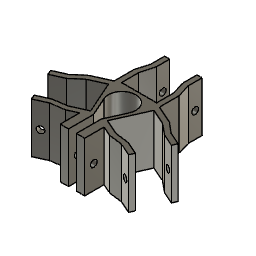
Battery Mount v1 (Autodesk Fusion 360 design; units mm, degrees)
Autodesk Fusion 360 part; units mm, degrees
note: some values were not read from the file. Set by a fixed rule: which sketch regions a step uses.
sketch "Sketch1" plane through (0, 0, 0) normal (0, 0, 1) x (1, 0, 0)
  line L0 (13.272, -15.3179) -> (7.3523, -12.6772)
  line L1 (22.727, -13.5264) -> (30.3778, -16.9328)
  line L2 (-18.8579, 11.9823) -> (-24.3388, 9.542)
  line L3 (-29.3341, 1.3169) -> (-26.7926, 3.4917)
  line L4 (10.5494, 15.7225) -> (10.5494, 25.9225)
  line L5 (-10.5507, 13.6692) -> (-12.6022, 13.6677)
  line L6 (-8.2853, 34.3148) -> (-10.558, 25.9259)
  line L7 (-22.9605, 6.8087) -> (-29.3341, 1.3169)
  line L8 (7.4982, 2.1403) -> (12.6022, 13.6692)
  line L9 (38.2942, 0.8476) -> (30.7617, 4.2012)
  line L10 (-18.8387, 11.9858) -> (-18.8579, 11.9823)
  line L11 (-13.6423, 10.9575) -> (-22.9605, 6.8087)
  line L12 (9.0778, 30.7724) -> (10.5494, 25.9225)
  line L13 (-13.6111, 26.0626) -> (-11.3383, 34.1084)
  line L14 (-36.985, -2.0895) -> (-29.3341, 1.3169)
  line L15 (37.0524, -1.9415) -> (29.7085, 1.3282)
  line L16 (30.7617, 4.2012) -> (24.3359, 9.5501)
  line L17 (-2.349, -24.3308) -> (-7.349, -24.3308)
  line L18 (13.607, 26.0699) -> (11.1789, 34.1274)
  line L19 (-24.3388, 9.542) -> (-30.7121, 4.0465)
  line L20 (-11.3383, 34.1084) -> (-13.6111, 26.0626)
  line L21 (-22.9605, 6.8087) -> (-13.6423, 10.9575)
  line L22 (30.3778, -16.9328) -> (29.1361, -19.7219)
  line L23 (-8.2853, 42.3537) -> (-11.3383, 42.3537)
  line L24 (37.0524, -1.9415) -> (38.2942, 0.8476)
  line L25 (2.3523, -24.3308) -> (7.3523, -24.3308)
  line L26 (-22.9665, -13.8111) -> (-14.3785, -12.4752)
  line L27 (-11.3383, 42.3537) -> (-8.2853, 42.3537)
  line L28 (-14.3785, -12.4752) -> (-22.9665, -13.8111)
  line L29 (-8.2853, 42.3537) -> (-8.2853, 34.3148)
  line L30 (7.3523, -12.6772) -> (7.3523, -24.3308)
  line L31 (8.1248, 33.9788) -> (9.0778, 30.7724)
  line L32 (11.1789, 34.1274) -> (13.607, 26.0699)
  line L33 (-2.349, -24.3308) -> (-2.349, -9.3308)
  line L34 (8.1248, 33.9788) -> (8.1248, 42.3537)
  line L35 (10.5494, 25.9225) -> (8.1248, 33.9788)
  line L36 (-10.5504, 15.7225) -> (-10.558, 25.9259)
  line L37 (-7.349, -24.3308) -> (-7.349, -12.6823)
  line L38 (-24.3388, 9.542) -> (-13.6024, 14.3172)
  line L39 (13.607, 26.0699) -> (13.6024, 14.3194)
  line L40 (-21.5362, -16.5162) -> (-29.0687, -19.8698)
  line L41 (7.7756, -12.8657) -> (7.7911, -12.8776)
  line L42 (22.9693, 6.8165) -> (29.7085, 1.3282)
  line L43 (24.3359, 9.5501) -> (14.8846, 13.7497)
  line L44 (29.7085, 1.3282) -> (22.9693, 6.8165)
  line L45 (13.6024, 20.0513) -> (13.607, 20.0703)
  line L46 (30.7617, 4.2012) -> (38.2942, 0.8476)
  line L47 (-21.5362, -16.5162) -> (-13.2615, -15.32)
  line L48 (13.272, -15.3179) -> (21.6205, -16.3769)
  line L49 (29.7085, 1.3282) -> (37.0524, -1.9415)
  line L50 (10.5494, 25.9225) -> (10.5494, 15.7225)
  line L51 (24.3359, 9.5501) -> (30.7617, 4.2012)
  line L52 (11.1778, 42.3537) -> (8.1248, 42.3537)
  line L53 (13.6024, 14.3194) -> (24.3359, 9.5501)
  line L54 (14.381, -12.4647) -> (22.727, -13.5264)
  line L55 (-12.6022, 13.6677) -> (-7.4976, 2.1397)
  line L56 (22.727, -13.5264) -> (19.4101, -13.0929)
  line L57 (30.3778, -16.9328) -> (22.727, -13.5264)
  line L58 (-38.2268, 0.6996) -> (-36.985, -2.0895)
  line L59 (-11.3383, 34.1084) -> (-11.3383, 42.3537)
  line L60 (19.4101, -13.0929) -> (14.381, -12.4647)
  line L61 (38.2942, 0.8476) -> (37.0524, -1.9415)
  line L62 (13.607, 20.0703) -> (13.607, 26.0699)
  line L63 (7.7911, -12.8776) -> (13.272, -15.3179)
  line L64 (-7.4976, 2.1397) -> (-2.349, -9.3308)
  line L65 (-13.6423, 10.9575) -> (-5.0603, -8.3182)
  line L66 (-11.3383, 42.3537) -> (-11.3383, 34.1084)
  line L67 (-8.2853, 34.3148) -> (-8.2853, 42.3537)
  line L68 (-29.3341, 1.3169) -> (-36.985, -2.0895)
  line L69 (-38.2268, 0.6996) -> (-30.7121, 4.0465)
  line L70 (-36.985, -2.0895) -> (-38.2268, 0.6996)
  line L71 (-26.7926, 3.4917) -> (-22.9605, 6.8087)
  line L72 (-30.7121, 4.0465) -> (-24.3388, 9.542)
  line L73 (-10.558, 25.9259) -> (-10.5504, 15.7225)
  line L74 (-13.2615, -15.32) -> (-21.5362, -16.5162)
  line L75 (14.381, -12.4647) -> (5.0628, -8.3159)
  line L76 (22.9693, 6.8165) -> (13.6449, 10.9597)
  line L77 (11.1778, 42.3537) -> (11.1789, 34.1274)
  line L78 (2.3523, -9.3308) -> (2.3523, -24.3308)
  line L79 (-10.558, 25.9259) -> (-8.2853, 34.3148)
  line L80 (8.1248, 42.3537) -> (8.1248, 33.9788)
  line L81 (5.0628, -8.3159) -> (14.381, -12.4647)
  line L82 (-7.349, -12.6823) -> (-13.2615, -15.32)
  line L83 (-5.0603, -8.3182) -> (-14.3785, -12.4752)
  line L84 (-7.349, -24.3308) -> (-2.349, -24.3308)
  line L85 (29.1361, -19.7219) -> (30.3778, -16.9328)
  line L86 (7.3523, -24.3308) -> (2.3523, -24.3308)
  line L87 (-14.3785, -12.4752) -> (-5.0603, -8.3182)
  line L88 (13.6449, 10.9597) -> (22.9693, 6.8165)
  line L89 (-30.3104, -17.0808) -> (-29.0687, -19.8698)
  line L90 (-29.0687, -19.8698) -> (-21.5362, -16.5162)
  line L91 (-29.0687, -19.8698) -> (-30.3104, -17.0808)
  line L92 (8.1248, 42.3537) -> (11.1778, 42.3537)
  line L93 (-2.349, -9.3308) -> (-2.349, -24.3308)
  line L94 (12.6022, 13.6692) -> (-10.5507, 13.6692)
  line L95 (10.5494, 15.7225) -> (-10.5504, 15.7225)
  arc A0 (7.4982, 2.1403) -> (-7.4976, 2.1397) centre (0.0002, 5.4599) ccw
  line L96 (2.3523, -9.3308) -> (7.4982, 2.1403)
  line L97 (-10.5504, 15.7225) -> (10.5494, 15.7225)
  line L98 (-5.0603, -8.3182) -> (-13.6423, 10.9575)
  line L99 (13.6449, 10.9597) -> (5.0628, -8.3159)
  line L100 (5.0628, -8.3159) -> (13.6449, 10.9597)
  circle A1 centre (0.0002, 5.4599) radius 8.2
  line L101 (21.6205, -16.3769) -> (29.1361, -19.7219)
  line L102 (-30.3104, -17.0808) -> (-22.9665, -13.8111)
  line L103 (-13.6111, 26.0626) -> (-13.6024, 14.3172)
  point P0 (0, 9)
  constraint coincident L23.end L27.start
  constraint coincident L23.start L27.end
  constraint coincident L6.start L29.end
  constraint coincident L6.end L36.end
  constraint coincident L36.start L73.end
  constraint coincident L4.start L50.end
  constraint coincident L4.end L12.end
  constraint coincident L31.start L34.start
  constraint coincident L34.end L52.end
  constraint coincident L52.start L77.start
  constraint coincident L18.end L32.start
  constraint coincident L18.start L32.end
  constraint coincident L16.end L43.start
  constraint coincident L9.end L16.start
  constraint coincident L9.start L24.end
  constraint coincident L15.start L24.start
  constraint coincident L15.end L42.end
  constraint coincident L42.start L44.end
  constraint coincident L76.end L88.start
  constraint coincident L75.end L81.start
  constraint coincident L54.start L60.end
  constraint coincident L1.start L54.end
  constraint coincident L1.end L22.start
  constraint coincident L22.end L85.start
  constraint coincident L0.start L48.start
  constraint coincident L25.end L30.end
  constraint coincident L25.start L78.end
  constraint coincident L78.start L96.start
  constraint coincident L8.start A0.start
  constraint coincident L55.end L64.start
  constraint coincident L33.end L64.end
  constraint coincident L17.start L33.start
  constraint coincident L17.end L37.start
  constraint coincident L47.end L74.start
  constraint coincident L40.start L47.start
  constraint coincident L40.end L89.end
  constraint coincident L89.start L91.end
  constraint coincident L26.start L28.end
  constraint coincident L26.end L28.start
  constraint coincident L65.end L83.start
  constraint coincident L11.start L21.end
  constraint coincident L7.start L11.end
  constraint coincident L3.start L7.end
  constraint coincident L14.start L58.end
  constraint coincident L58.start L69.start
  constraint coincident L19.end L69.end
  constraint coincident L2.end L19.start
  constraint coincident L13.start L20.end
  constraint coincident L13.end L20.start
  constraint concentric A0 A1
  constraint collinear L84 L86
  constraint perpendicular L91 L102
extrude "Extrude1" add sketch "Sketch1" along normal blind 30 contours L0 L1 L4 L5 L6 L7 L8 L9 L11 L13 L14 L15 L16 L17 L18 L19 L20 L21 L22 L23 L24 L25 L26 L27 L28 L29 L30 L32 L33 L34 L35 L36 L37 L38 L39 L40 L42 L43 L44 L46 L47 L48 L49 L50 L51 L52 L53 L54 L55 L57 L58 L59 L61 L64 L65 L66 L67 L68 L69 L70 L72 L73 L74 L75 L76 L77 L78 L79 L80 L81 L82 L83 L84 L85 L86 L87 L88 L89 L90 L91 L92 L93 L94 L95 L96 L97 L98 L99 L100 L101 L102 L103 | L5 L8 L55 L94 A0 A1
sketch "Sketch2" plane through (2.5741, -5.7816, 0) normal (0.406737, -0.913545, 0) x (0.913545, 0.406737, 0)
  line L0 (-34.6373, 0) -> (-26.392, 0)
  line L1 (-26.392, 0) -> (-26.392, 30)
  line L2 (-26.392, 30) -> (-34.6373, 30)
  line L3 (-34.6373, 30) -> (-34.6373, 0)
  line L4 (-34.6373, 30) -> (-26.392, 0) construction
  line L5 (-34.6373, 0) -> (-26.392, 30) construction
  circle A0 centre (-30.5147, 15) radius 2
  dimension "d3" = 4
  constraint coincident L2.end L3.start
  constraint coincident L0.end L1.start
  constraint coincident L0.start L3.end
  constraint coincident L1.end L2.start
  constraint midpoint L5 A0.centre
  measures "d3" diameter of A0
extrude "Extrude2" cut sketch "Sketch2" against normal blind 23 contours A0
sketch "Sketch3" plane through (-11.3383, 0, 0) normal (-1, 0, 0) x (0, -1, 0)
  line L0 (-42.3537, 0) -> (-34.1084, 0)
  line L1 (-34.1084, 0) -> (-34.1084, 30)
  line L2 (-34.1084, 30) -> (-42.3537, 30)
  line L3 (-42.3537, 30) -> (-42.3537, 0)
  line L4 (-42.3537, 30) -> (-34.1084, 0) construction
  line L5 (-42.3537, 0) -> (-34.1084, 30) construction
  circle A0 centre (-38.2311, 15) radius 2
  dimension "d6" = 4
  constraint coincident L2.end L3.start
  constraint coincident L0.end L1.start
  constraint coincident L0.start L3.end
  constraint coincident L1.end L2.start
  constraint midpoint L4 A0.centre
  measures "d6" diameter of A0
extrude "Extrude3" cut sketch "Sketch3" against normal blind 23 contours A0
sketch "Sketch4" plane through (6.6501, 14.9364, 0) normal (0.406737, 0.913545, 0) x (-0.913545, 0.406737, 0)
  line L0 (-34.6387, 0) -> (-26.3934, 0)
  line L1 (-26.3934, 0) -> (-26.3934, 30)
  line L2 (-26.3934, 30) -> (-34.6387, 30)
  line L3 (-34.6387, 30) -> (-34.6387, 0)
  line L4 (-34.6387, 30) -> (-26.3934, 0) construction
  line L5 (-34.6387, 0) -> (-26.3934, 30) construction
  circle A0 centre (-30.5161, 15) radius 2
  dimension "d9" = 4
  constraint coincident L2.end L3.start
  constraint coincident L0.end L1.start
  constraint coincident L0.start L3.end
  constraint coincident L1.end L2.start
  constraint midpoint L4 A0.centre
  measures "d9" diameter of A0
extrude "Extrude4" cut sketch "Sketch4" against normal blind 24 contours A0
sketch "Sketch5" plane through (7.3523, 0, 0) normal (1, 0, 0) x (0, 1, 0)
  line L0 (-24.3308, 0) -> (-12.6772, 0)
  line L1 (-12.6772, 0) -> (-12.6772, 30)
  line L2 (-12.6772, 30) -> (-24.3308, 30)
  line L3 (-24.3308, 30) -> (-24.3308, 0)
  line L4 (-24.3308, 30) -> (-14, 0) construction
  line L5 (-24.3308, 0) -> (-12.6772, 30) construction
  circle A0 centre (-18.8546, 14.0974) radius 2
  dimension "d12" = 4
  constraint coincident L2.end L3.start
  constraint coincident L0 L4.end
  constraint coincident L0.start L3.end
  constraint coincident L1.end L2.start
  constraint coincident L5 A0.centre
  constraint coincident L4 A0.centre
  measures "d12" diameter of A0
extrude "Extrude5" cut sketch "Sketch5" against normal blind 17 contours A0
